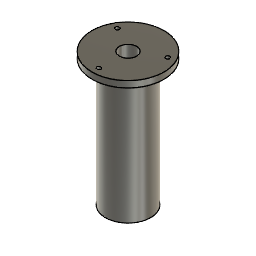
charing_dock_leg (Autodesk Fusion 360 design; units mm, degrees)
part number: 2026-05-25-11-58-39-104
Autodesk Fusion 360 part; units mm, degrees
sketch "Sketch1" plane through (0, 0, 0) normal (0, 0, 1) x (1, 0, 0)
  circle A0 centre (0, 0) radius 17.855
  circle A1 centre (0, 0) radius 6.75
  dimension "d1" = 35.71
  dimension "d2" = 13.5
  constraint coincident A0.centre A1.centre
  constraint concentric A0 A1
  measures "d1" diameter of A0
  measures "d2" diameter of A1
extrude "Extrude1" add sketch "Sketch1" along normal blind 100
sketch "Sketch2" plane through (0, 0, 0) normal (0, 0, -1) x (1, 0, 0)
  circle A0 centre (0, 0) radius 6.75
  circle A1 centre (0, 0) radius 17.855
  circle A2 centre (0.2482, -12.264) radius 1.4
  circle A3 centre (10.5133, 5.8699) radius 1.4
  circle A4 centre (-10.3222, 5.8177) radius 1.4
  dimension "d5" = 2.8
  dimension "d6" = 2.8
  dimension "d7" = 2.8
  measures "d5" diameter of A2
  measures "d6" diameter of A3
  measures "d7" diameter of A4
extrude "Extrude2" cut sketch "Sketch2" against normal blind 13 contours A2 | A3 | A4
sketch "Sketch3" plane through (0, 0, 100) normal (0, 0, 1) x (1, 0, 0)
  circle A0 centre (0, 0) radius 28.439
  circle A1 centre (0, 0) radius 6.75
  circle A2 centre (0, 0) radius 17.855
  constraint coincident A0.centre A1.centre
extrude "Extrude3" add sketch "Sketch3" along normal blind 5 contours A0 | A2
sketch "Sketch4" plane through (0, 0, 100) normal (0, 0, -1) x (1, 0, 0)
  circle A0 centre (0, 0) radius 28.439
  circle A1 centre (0, 0) radius 17.855
  circle A2 centre (0, 23.0024) radius 1.6
  circle A3 centre (-19.9207, -11.5012) radius 1.6
  circle A4 centre (19.9207, -11.5012) radius 1.6
  dimension "d17" = 3.2
  dimension "d19" = 360
  measures "d17" diameter of A2
extrude "Extrude4" cut sketch "Sketch4" against normal blind 5 contours A2 | A3 | A4
